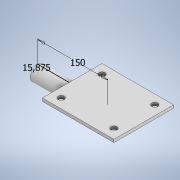
# Autodesk Inventor part: Spindle
Saved by Autodesk Inventor 2020 (Build 240168000, 168)
## iProperties
Created: 2020-03-12
Part Number: Spindle
Material: Generic
Document SubType Name: Modeling
Designer: jgranlund
Density: 1 g/cm^3
Appearance: Default
Author: jgranlund
Autodesk Inventor part; units mm, degrees
ref_plane "YZ Plane" through (0, 0, 0) normal (1, 0, 0) x (0, 1, 0)
ref_plane "XZ Plane" through (0, 0, 0) normal (0, 1, 0) x (-1, 0, 0)
ref_plane "XY Plane" through (0, 0, 0) normal (0, 0, 1) x (1, 0, 0)
sketch "Sketch1" plane through (0, 0, 0) normal (0, 0, 1) x (1, 0, 0)
  line L0 (0, 0) -> (-150, 0)
  line L1 (-150, 0) -> (-150, 15.875)
  line L2 (-150, 15.875) -> (0, 15.875)
  line L3 (0, 15.875) -> (0, 0)
  dimension "d0" = 150
  dimension "d1" = 15.875
  constraints: 8 end point, 3 perpendicular, 1 horizontal
  measures "d0" distance of L1.end L2.end
  measures "d1" distance of L0.end L1.end
revolve "Revolution1" add sketch "Sketch1" angle 360 about axis through (0, 0, 0) along (-1, 0, 0)
sketch "Sketch2" plane through (0, 0, 0) normal (1, 0, 0) x (0, 0, -1)
  circle A0 centre (0, 0) radius 15.875 projected
  line L0 (0, 15.875) -> (-63.5, 15.875)
  line L1 (0, 15.875) -> (63.5, 15.875)
  line L2 (0, 15.875) -> (-63.5, 15.875) construction
  line L3 (0, 15.875) -> (63.5, 15.875) construction
  line L4 (-63.5, 15.875) -> (-63.5, 22.225)
  line L5 (-63.5, 22.225) -> (63.5, 22.225)
  line L6 (63.5, 22.225) -> (63.5, 15.875)
  dimension "d3" = 63.5
  dimension "d5" = 6.35
  constraints: 14 end point, 4 horizontal, 3 collinear, 1 parallel, 1 perpendicular, 1 point on line, 1 vertical, 1 vertical alignment, 1 other
  measures "d3" distance of L0.start L0.end
  measures "d5" distance of L0.end L4.end
extrude "Extrusion1" add sketch "Sketch2" along normal mid plane 152.4 contours L0 L4 L5 L6 L1
sketch "Sketch3" plane through (-76.2, 22.225, 63.5) normal (0, 1, 0) x (1, 0, 0)
  circle A0 centre (20, 107) radius 6.5
  circle A1 centre (132.4, 107) radius 6.5
  circle A2 centre (132.4, 20) radius 6.5
  circle A3 centre (20, 20) radius 6.5
  line L0 (0, 0) -> (0, 127) projected
  line L1 (0, 127) -> (152.4, 127) projected
  line L2 (20, 107) -> (0, 107) construction
  line L3 (20, 107) -> (20, 127) construction
  line L4 (152.4, 127) -> (0, 127) construction
  line L5 (132.4, 107) -> (132.4, 127) construction
  line L6 (132.4, 107) -> (152.4, 107) construction
  line L7 (152.4, 127) -> (152.4, 0) construction
  line L8 (20, 20) -> (0, 20) construction
  line L9 (20, 20) -> (20, 0) construction
  line L10 (0, 0) -> (152.4, 0) construction
  line L11 (132.4, 20) -> (152.4, 20) construction
  line L12 (132.4, 20) -> (132.4, 0) construction
  point P0 (76.2, 63.5)
  dimension "d8" = 13
  dimension "d9" = 13
  dimension "d10" = 13
  dimension "d11" = 13
  dimension "d16" = 20
  constraints: 16 end point, 8 point on line, 7 equal length, 5 perpendicular, 4 centre point, 3 horizontal
  measures "d8" diameter of A0
  measures "d9" diameter of A1
  measures "d10" diameter of A2
  measures "d11" diameter of A3
  measures "d16" distance of L2.start L2.end
extrude "Extrusion2" cut sketch "Sketch3" against normal through all
body "Solid1"
